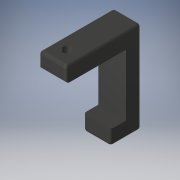
# Autodesk Inventor part: bed_spring_holder_front
Saved by Autodesk Inventor 2018 (Build 220112000, 112)
## iProperties
Created: 2018-05-25
Part Number: bed_spring_holder_front
Material: Plastic, Opaque Black
Document SubType Name: Modeling
Designer: Z. Deniz
Density: 0.952 g/cm^3
Appearance: Smooth - Black
Author: Z. Deniz
Autodesk Inventor part; units mm, degrees
ref_plane "YZ Plane" through (0, 0, 0) normal (1, 0, 0) x (0, 1, 0)
ref_plane "XZ Plane" through (0, 0, 0) normal (0, 1, 0) x (-1, 0, 0)
ref_plane "XY Plane" through (0, 0, 0) normal (0, 0, 1) x (1, 0, 0)
sketch "Sketch1" plane through (0, 0, 0) normal (1, 0, 0) x (0, 1, 0)
  line L0 (0, 0) -> (30, 0)
  line L1 (30, 0) -> (30, 24.5)
  line L2 (30, 24.5) -> (25, 24.5)
  line L3 (25, 24.5) -> (25, 5)
  line L4 (25, 5) -> (5, 5)
  line L5 (5, 5) -> (5, 10)
  line L6 (5, 10) -> (0, 10)
  line L7 (0, 10) -> (0, 0)
  line L8 (25, 5) -> (32.5, 5) construction
  dimension "d0" = 30
  dimension "d1" = 24.5
  dimension "d2" = 5
  dimension "d3" = 19.5
  dimension "d9" = 5
  dimension "d10" = 5
  constraints: 18 end point, 6 perpendicular, 2 horizontal, 1 point on line, 1 vertical
  measures "d0" distance of L0.start L0.end
  measures "d1" distance of L0.end L1.end
  measures "d2" distance of L1.end L2.end
  measures "d3" distance of L2.end L3.end
  measures "d9" distance of L4.end L5.end
  measures "d10" distance of L5.end L6.end
extrude "Extrusion1" add sketch "Sketch1" along normal blind 9
sketch "Sketch4" plane through (0, 30, 24.5) normal (0, 1, 0) x (1, 0, 0)
  circle A0 centre (4.5, 5) radius 1.575
  line L0 (0, 0) -> (9, 0) projected
  line L1 (0, 24.5) -> (0, 0) projected
  dimension "d18" = 3.15
  dimension "d19" = 5
  dimension "d20" = 4.5
  constraints: 1 centre point
  measures "d18" diameter of A0
  measures "d19" distance from line of L0 A0.centre
  measures "d20" distance from line of A0.centre L1
extrude "Extrusion3" cut sketch "Sketch4" against normal blind 5
fillet "Fillet1" radius 1 15 edges at (9, 0, 5) (4.5, 0, 10) (0, 0, 5) (4.5, 0, 0) (9, 15, 0) (0, 15, 0) (9, 30, 12.25) (4.5, 30, 0) (0, 30, 12.25) (4.5, 30, 24.5) (4.5, 25, 24.5) (9, 27.5, 24.5) (0, 27.5, 24.5) (9, 2.5, 10) (0, 2.5, 10)
body "Solid1"
